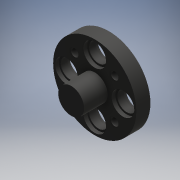
# Autodesk Inventor part: xl320_wheel
Saved by Autodesk Inventor 2016 (Build 200138000, 138)
## iProperties
Created: 2016-04-30
Part Number: xl320_wheel
Material: PC/ABS Plastic
Document SubType Name: Modeling
Designer: Ali
Density: 0.357273 g/cm^3
Appearance: Smooth - Light Gray
Author: Ali
Autodesk Inventor part; units mm, degrees
ref_plane "YZ Plane" through (0, 0, 0) normal (1, 0, 0) x (0, 1, 0)
ref_plane "XZ Plane" through (0, 0, 0) normal (0, 1, 0) x (-1, 0, 0)
sketch "Sketch1" plane through (0, 0, 0) normal (0, 1, 0) x (-1, 0, 0)
  circle A0 centre (0, 0) radius 8.825
  dimension "d0" = 17.65
  constraints: 1 centre point, 1 coincident
  measures "d0" diameter of A0
extrude "Extrusion1" add sketch "Sketch1" along normal blind 3
sketch "Sketch2" plane through (0, 0, 0) normal (0, -1, 0) x (1, 0, 0)
  circle A0 centre (0, 0) radius 8.825 projected
  circle A1 centre (0, 0) radius 2.75
  dimension "d3" = 5.5
  constraints: 1 centre point, 1 coincident
  measures "d3" diameter of A1
extrude "Extrusion2" add sketch "Sketch2" along normal blind 5 contours A1
sketch "Sketch3" plane through (0, 3, 0) normal (0, 1, 0) x (1, 0, 0)
  circle A0 centre (0, 0) radius 8.825 projected
  circle A1 centre (-6, 0) radius 2
  line L0 (-6, 0) -> (5.0545, 0) construction
  circle A2 centre (0, -6) radius 2
  circle A3 centre (6, 0) radius 2
  circle A4 centre (0, 6) radius 2
  circle A5 centre (-4.2426, 4.2426) radius 0.8
  line L1 (0, 0) -> (-4.2426, 4.2426) construction
  circle A6 centre (0, 0) radius 2.75 projected
  arc A7 (0, 6) -> (-6, 0) centre (0, 0) ccw construction
  circle A8 centre (-4.2426, -4.2426) radius 0.8
  circle A9 centre (4.2426, -4.2426) radius 0.8
  circle A10 centre (4.2426, 4.2426) radius 0.8
  dimension "d6" = 4
  dimension "d7" = 6
  dimension "d10" = 360
  dimension "d14" = 1.6
  dimension "d15" = 45
  dimension "d18" = 360
  constraints: 9 centre point, 4 end point, 3 point on circle, 1 coincident, 1 horizontal, 1 point on line, 18 other
  measures "d6" diameter of A1
  measures "d7" distance of L0.start L1.start
  measures "d14" diameter of A5
  measures "d15" angle of L1 L0
extrude "Extrusion3" cut sketch "Sketch3" against normal through all contours A1 | A2 | A3 | A4 | A5 | A8 | A9 | A10
sketch "Sketch4" plane through (0, 3, 0) normal (0, 1, 0) x (1, 0, 0)
  circle A0 centre (6, 0) radius 2 projected
  circle A1 centre (-6, 0) radius 2 projected
  circle A2 centre (0, -6) radius 2 projected
  circle A3 centre (0, 6) radius 2 projected
  circle A4 centre (0, 6) radius 2.4
  circle A5 centre (-6, 0) radius 2.4
  circle A6 centre (6, 0) radius 2.4
  circle A7 centre (0, -6) radius 2.4
  dimension "d20" = 0.4
  dimension "d21" = 0.4
  dimension "d22" = 0.4
  dimension "d23" = 0.4
  constraints: 4 centre point
  measures "d20" radial gap between concentric circles of A3 A4
  measures "d21" radial gap between concentric circles of A1 A5
  measures "d22" radial gap between concentric circles of A0 A6
  measures "d23" radial gap between concentric circles of A2 A7
extrude "Extrusion4" cut sketch "Sketch4" against normal blind 0.8
ref_plane "Work Plane1" through (0, 1.5, 0) normal (0, 1, 0) x (1, 0, 0)
mirror "Mirror1" about plane through (0, 1.5, 0) normal (0, 1, 0) of "Extrusion4"
body "Solid1"
